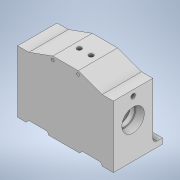
# Autodesk Inventor part: 731113
Saved by Autodesk Inventor 2022 (Build 260153000, 153)
## iProperties
Created: 2021-10-26
Part Number: 731113
Material: Типовые
Document SubType Name: Modeling
Designer: RaNSiD
Density: 1 g/cm^3
Appearance: По умолчанию
Author: RaNSiD
Autodesk Inventor part; units mm, degrees
ref_plane "YZ Plane" through (0, 0, 0) normal (1, 0, 0) x (0, 1, 0)
ref_plane "XZ Plane" through (0, 0, 0) normal (0, 1, 0) x (-1, 0, 0)
ref_plane "XY Plane" through (0, 0, 0) normal (0, 0, 1) x (1, 0, 0)
sketch "Эскиз1" plane through (0, 0, 0) normal (0, 0, 1) x (1, 0, 0)
  line L0 (0, 0) -> (170, 0)
  line L1 (170, 0) -> (170, 110)
  line L2 (170, 110) -> (150, 110)
  line L3 (0, 110) -> (0, 0)
  line L4 (20, 110) -> (62.5, 125.4687)
  line L5 (62.5, 125.4687) -> (107.5, 125.4687)
  line L6 (107.5, 125.4687) -> (150, 110)
  line L7 (20, 110) -> (0, 110)
  dimension "d0" = 170
  dimension "d1" = 110
  dimension "d3" = 45
  dimension "d4" = 160
  dimension "d5" = 160
  dimension "d6" = 20
  constraints: 16 end point, 3 parallel, 2 equal length, 2 horizontal, 1 perpendicular
  measures "d0" distance of L3.start L1.end
  measures "d1" distance of L1.end L0.end
  measures "d3" distance of L4.end L5.end
  measures "d4" angle of L7 L4
  measures "d5" angle of L2 L6
  measures "d6" distance of L4.start L3.start
extrude "Выдавливание1" add sketch "Эскиз1" along normal mid plane 70
sketch "Эскиз2" plane through (0, 0, 35) normal (-1, 0, 0) x (0, 0, 1)
  line L0 (-70, 0) -> (-87, 0)
  line L1 (-87, 0) -> (-87, 10)
  line L2 (-87, 10) -> (-70, 10)
  line L3 (-70, 10) -> (-70, 0)
  point P0 (-35, 0)
  dimension "d9" = 17
  dimension "d10" = 10
  constraints: 8 end point, 2 parallel, 1 horizontal, 1 perpendicular
  measures "d9" distance of L1.end L2.end
  measures "d10" distance of L0.end L1.end
extrude "Выдавливание2" add sketch "Эскиз2" against normal blind 170
fillet "Сопряжение1" radius 7 1 edges at (85, 10, -35)
sketch "Эскиз3" plane through (0, 0, 35) normal (0, 0, 1) x (1, 0, 0)
  line L0 (0, 0) -> (170, 0) construction
  line L1 (20, 0) -> (55, 0)
  line L2 (55, 0) -> (55, 5)
  line L3 (55, 5) -> (20, 5)
  line L4 (20, 5) -> (20, 0)
  line L5 (115, 0) -> (150, 0)
  line L6 (150, 0) -> (150, 5)
  line L7 (150, 5) -> (115, 5)
  line L8 (115, 5) -> (115, 0)
  line L9 (20, 5) -> (0, 5) construction
  line L10 (0, 110) -> (0, 0) construction
  line L11 (115, 5) -> (55, 5) construction
  line L12 (150, 5) -> (170, 5) construction
  line L13 (170, 0) -> (170, 110) construction
  dimension "d14" = 35
  dimension "d15" = 5
  dimension "d16" = 35
  dimension "d17" = 5
  dimension "d18" = 20
  constraints: 22 end point, 5 point on line, 4 parallel, 3 horizontal, 2 perpendicular, 1 collinear
  measures "d14" distance of L3.end L2.end
  measures "d15" distance of L2.end L1.end
  measures "d16" distance of L7.end L6.end
  measures "d17" distance of L6.end L5.end
  measures "d18" distance of L6.end L12.end
extrude "Выдавливание3" cut sketch "Эскиз3" against normal through all
fillet "Сопряжение2" radius 5 2 edges at (150, 5, -8.5) (55, 5, -8.5)
chamfer "Фаска1" distance 5 angle 45 2 edges at (20, 0, -8.5) (115, 0, -8.5)
sketch "Эскиз4" plane through (0, 0, 35) normal (-1, 0, 0) x (0, 0, 1)
  line L0 (0, 110) -> (-70, 110) construction
  point P0 (-35, 0)
  point P1 (-35, 100)
  dimension "d25" = 10
  constraints: 1 vertical alignment
  measures "d25" distance from line of L0 point (-35, 100)
hole "Отверстие1" at (0, 100, 0) direction (1, 0, 0) diameter 8 end through all
sketch "Эскиз5" plane through (62.5, 125.4687, 35) normal (0, 1, 0) x (1, 0, 0)
  line L0 (0, 70) -> (0, 0) construction
  line L1 (45, 70) -> (45, 0) construction
  point P0 (-62.5, 35)
  point P1 (12, 35)
  point P2 (33, 35)
  dimension "d33" = 12
  dimension "d34" = 12
  constraints: 2 horizontal alignment
  measures "d33" distance from line of L0 point (12, 35)
  measures "d34" distance from line of L1 point (33, 35)
hole "Отверстие2" at (74.5, 125.4687, 0) at (95.5, 125.4687, 0) direction (0, -1, 0) diameter 8 depth 34
sketch "Эскиз6" plane through (0, 0, 35) normal (0, 0, 1) x (1, 0, 0)
  line L0 (70.5, 125.4687) -> (78.5, 125.4687) projected
  line L1 (91.5, 125.4687) -> (99.5, 125.4687) projected
  line L2 (0, 96) -> (0, 104) projected
  line L3 (170, 104) -> (170, 96) projected
  line L4 (107.5, 125.4687) -> (62.5, 125.4687) projected
  point P0 (0, 0)
  point P1 (62.5, 119.4687)
  point P2 (107.5, 119.4687)
  dimension "d42" = 6
  constraints: 2 vertical alignment, 1 horizontal alignment
  measures "d42" distance from line of L4 point (107.5, 119.469)
hole "Отверстие3" at (62.5, 119.4687, 35) at (107.5, 119.4687, 35) direction (0, 0, -1) diameter 5 end through all
sketch "Эскиз7" plane through (0, 0, 0) normal (0, 0, 1) x (1, 0, 0)
  line L0 (0, 17) -> (0, 110) construction
  line L1 (0, 63.5) -> (170, 63.5)
  line L2 (170, 110) -> (170, 17) construction
  line L3 (0, 83.5) -> (15, 83.5)
  line L4 (0, 63.5) -> (0, 83.5)
  line L5 (15, 83.5) -> (15, 81.5)
  line L6 (15, 81.5) -> (23, 81.5)
  line L7 (23, 81.5) -> (25, 83.5)
  line L8 (62.5, 125.4687) -> (107.5, 125.4687) construction
  line L9 (55, 0) -> (110, 0) projected
  line L10 (85, 125.4687) -> (85, 0) construction
  line L11 (170, 83.5) -> (155, 83.5)
  line L12 (170, 63.5) -> (170, 83.5)
  line L13 (155, 83.5) -> (155, 81.5)
  line L14 (155, 81.5) -> (147, 81.5)
  line L15 (147, 81.5) -> (145, 83.5)
  line L16 (145, 83.5) -> (145, 78.5)
  line L17 (145, 78.5) -> (142.1716, 75.6716)
  line L18 (142.1716, 75.6716) -> (133.1716, 75.6716)
  line L19 (133.1716, 75.6716) -> (130.3431, 78.5)
  line L20 (130.3431, 78.5) -> (130.3431, 83.5)
  line L21 (130.3431, 83.5) -> (122.3431, 83.5)
  line L22 (145, 83.5) -> (145, 78.5)
  line L23 (145, 78.5) -> (142.1716, 75.6716)
  line L24 (142.1716, 75.6716) -> (133.1716, 75.6716)
  line L25 (133.1716, 75.6716) -> (130.3431, 78.5)
  line L26 (130.3431, 78.5) -> (130.3431, 83.5)
  line L27 (130.3431, 83.5) -> (122.3431, 83.5)
  line L28 (122.3431, 83.5) -> (122.3431, 78.5)
  line L29 (122.3431, 78.5) -> (119.5147, 75.6716)
  line L30 (119.5147, 75.6716) -> (110.5147, 75.6716)
  line L31 (110.5147, 75.6716) -> (107.6863, 78.5)
  line L32 (107.6863, 78.5) -> (107.6863, 83.5)
  line L33 (107.6863, 83.5) -> (99.6863, 83.5)
  line L34 (99.6863, 83.5) -> (99.6863, 78.5)
  line L35 (99.6863, 78.5) -> (96.8579, 75.6716)
  line L36 (96.8579, 75.6716) -> (87.8579, 75.6716)
  line L37 (87.8579, 75.6716) -> (85.0294, 78.5)
  line L38 (85.0294, 78.5) -> (85.0294, 83.5)
  line L39 (85.0294, 83.5) -> (77.0294, 83.5)
  line L40 (77.0294, 83.5) -> (77.0294, 78.5)
  line L41 (77.0294, 78.5) -> (74.201, 75.6716)
  line L42 (74.201, 75.6716) -> (65.201, 75.6716)
  line L43 (65.201, 75.6716) -> (62.3726, 78.5)
  line L44 (62.3726, 78.5) -> (62.3726, 83.5)
  line L45 (62.3726, 83.5) -> (54.3726, 83.5)
  line L46 (62.3726, 83.5) -> (54.3726, 83.5)
  line L47 (62.3726, 78.5) -> (62.3726, 83.5)
  line L48 (65.201, 75.6716) -> (62.3726, 78.5)
  line L49 (74.201, 75.6716) -> (65.201, 75.6716)
  line L50 (77.0294, 78.5) -> (74.201, 75.6716)
  line L51 (77.0294, 83.5) -> (77.0294, 78.5)
  line L52 (39.7157, 83.5) -> (25, 83.5)
  line L53 (39.7157, 78.5) -> (39.7157, 83.5)
  line L54 (42.5442, 75.6716) -> (39.7157, 78.5)
  line L55 (51.5442, 75.6716) -> (42.5442, 75.6716)
  line L56 (54.3726, 78.5) -> (51.5442, 75.6716)
  line L57 (54.3726, 83.5) -> (54.3726, 78.5)
  line L58 (25, 83.5) -> (25, 63.5)
  line L59 (145, 83.5) -> (145, 63.5)
  point P0 (0, 0)
  dimension "d52" = 2
  dimension "d54" = 135
  dimension "d55" = 8
  dimension "d84" = 40
  dimension "d85" = 25
  dimension "d86" = 5
  dimension "d87" = 4
  dimension "d88" = 135
  dimension "d89" = 9
  dimension "d90" = 4
  dimension "d91" = 8
  dimension "d92" = 5
  dimension "d93" = 4
  dimension "d94" = 135
  dimension "d95" = 9
  dimension "d96" = 4
  dimension "d97" = 8
  dimension "d98" = 5
  dimension "d99" = 4
  dimension "d100" = 135
  dimension "d101" = 9
  dimension "d102" = 4
  dimension "d103" = 8
  dimension "d104" = 5
  dimension "d105" = 4
  dimension "d106" = 135
  dimension "d107" = 9
  dimension "d108" = 4
  dimension "d109" = 8
  dimension "d110" = 5
  dimension "d111" = 4
  dimension "d112" = 135
  dimension "d113" = 9
  dimension "d114" = 4
  dimension "d115" = 8
  dimension "d116" = 5
  dimension "d117" = 4
  dimension "d118" = 135
  dimension "d119" = 9
  dimension "d120" = 4
  dimension "d121" = 8
  dimension "d122" = 5
  dimension "d123" = 4
  dimension "d124" = 135
  dimension "d125" = 9
  constraints: 112 end point, 25 perpendicular, 14 parallel, 8 vertical, 5 symmetric about line, 4 point on line, 3 midpoint, 1 horizontal, 1 horizontal alignment
  measures "d52" distance of L3.end L5.end
  measures "d54" angle of L3 L7
  measures "d55" distance of L5.end L6.end
  measures "d84" diameter of L3 L1
  measures "d85" distance of L3.start L7.end
  measures "d86" distance of L15.end L16.end
  measures "d87" distance of L16.end L17.end
  measures "d88" angle of L16 L17
  measures "d89" distance of L17.end L18.end
  measures "d90" distance of L18.end L19.end
  measures "d91" distance of L20.end L21.end
  measures "d92" distance of L15.end L23.start
  measures "d93" distance of L23.start L24.start
  measures "d94" angle of L22 L23
  measures "d95" distance of L24.start L25.start
  measures "d96" distance of L25.start L26.start
  measures "d97" distance of L27.start L27.end
  measures "d98" distance of L21.end L29.start
  measures "d99" distance of L29.start L30.start
  measures "d100" angle of L28 L29
  measures "d101" distance of L30.start L31.start
  measures "d102" distance of L31.start L32.start
  measures "d103" distance of L33.start L33.end
  measures "d104" distance of L33.end L35.start
  measures "d105" distance of L35.start L36.start
  measures "d106" angle of L34 L35
  measures "d107" distance of L36.start L37.start
  measures "d108" distance of L37.start L38.start
  measures "d109" distance of L39.end L39.start
  measures "d110" distance of L39.end L41.start
  measures "d111" distance of L41.start L42.start
  measures "d112" angle of L40 L41
  measures "d113" distance of L42.start L43.start
  measures "d114" distance of L43.start L44.start
  measures "d115" distance of L45.start L45.end
  measures "d116" distance of L39.end L50.start
  measures "d117" distance of L50.start L49.start
  measures "d118" angle of L51 L50
  measures "d119" distance of L49.start L48.start
  measures "d120" distance of L48.start L47.start
  measures "d121" distance of L46.start L46.end
  measures "d122" distance of L45.end L56.start
  measures "d123" distance of L56.start L55.start
  measures "d124" angle of L57 L56
  measures "d125" distance of L55.start L54.start
revolve "Вращение2" cut sketch "Эскиз7" angle 360 about axis through (0, 63.5, 0) along (1, 0, 0) contours L4 L3 L5 L6 L7 L58 L1 | L59 L16 L15 L14 L13 L11 L12 L1
sketch "Эскиз9" plane through (0, 0, 0) normal (0, 0, 1) x (1, 0, 0)
  line L0 (25, 83.5) -> (25, 43.5) construction
  line L1 (25, 43.5) -> (145, 43.5)
  line L2 (145, 43.5) -> (145, 15)
  line L3 (145, 15) -> (91.8199, 15)
  line L4 (25, 15) -> (25, 43.5)
  line L5 (145, 83.5) -> (145, 43.5) construction
  line L6 (50, 5) -> (20, 5) construction
  line L7 (73.1801, 15) -> (75, 10)
  line L8 (75, 10) -> (90, 10)
  line L9 (0, 17) -> (170, 17) construction
  line L10 (90, 10) -> (91.8199, 15)
  line L11 (73.1801, 15) -> (25, 15)
  line L12 (55, 0) -> (110, 0) construction
  point P0 (0, 0)
  point P1 (145, 63.5)
  point P2 (82.5, 10)
  point P3 (82.5, 0)
  dimension "d178" = 110
  dimension "d179" = 110
  dimension "d180" = 15
  dimension "d181" = 5
  dimension "d182" = 10
  constraints: 16 end point, 4 parallel, 3 midpoint, 2 vertical alignment, 1 horizontal, 1 horizontal alignment, 1 perpendicular
  measures "d178" angle of L8 L10
  measures "d179" angle of L8 L7
  measures "d180" distance of L7.end L8.end
  measures "d181" distance between parallel lines of L3 L8
  measures "d182" distance between parallel lines of L6 L11
extrude "Выдавливание4" cut sketch "Эскиз9" along normal mid plane 15
sketch "Эскиз10" plane through (75, 10, -7.5) normal (0, 1, 0) x (1, 0, 0)
  line L0 (15, 0) -> (0, 0) construction
  line L1 (15, 0) -> (15, -15) construction
  point P0 (-75, -7.5)
  point P1 (7.5, -7.5)
  point P2 (7.5, 0)
  point P3 (15, -7.5)
  constraints: 2 midpoint, 1 horizontal alignment, 1 vertical alignment
hole "Отверстие4" at (82.5, 10, 0) direction (0, -1, 0) diameter 12 end through all
sketch "Эскиз11" plane through (0, 0, 0) normal (0, 0, 1) x (1, 0, 0)
  line L0 (0, 17) -> (0, 110) construction
  line L1 (0, 63.5) -> (170, 63.5)
  line L2 (170, 127) -> (170, 0) construction
  line L3 (0, 83.5) -> (15, 83.5)
  line L4 (0, 63.5) -> (0, 83.5)
  line L5 (15, 83.5) -> (15, 81.5)
  line L6 (15, 81.5) -> (23, 81.5)
  line L7 (23, 81.5) -> (25, 83.5)
  line L8 (62.5, 125.4687) -> (107.5, 125.4687) construction
  line L9 (55, 0) -> (110, 0) construction
  line L10 (85, 125.4687) -> (85, 0) construction
  line L11 (147, 81.5) -> (145, 83.5)
  line L12 (155, 81.5) -> (147, 81.5)
  line L13 (155, 83.5) -> (155, 81.5)
  line L14 (170, 83.5) -> (155, 83.5)
  line L15 (170, 63.5) -> (170, 83.5)
  line L16 (145, 83.5) -> (145, 78.5)
  line L17 (145, 78.5) -> (142.1716, 75.6716)
  line L18 (142.1716, 75.6716) -> (133.1716, 75.6716)
  line L19 (133.1716, 75.6716) -> (130.3431, 78.5)
  line L20 (130.3431, 78.5) -> (130.3431, 83.5)
  line L21 (130.3431, 83.5) -> (122.3431, 83.5)
  line L22 (130.3431, 83.5) -> (122.3431, 83.5)
  line L23 (130.3431, 78.5) -> (130.3431, 83.5)
  line L24 (133.1716, 75.6716) -> (130.3431, 78.5)
  line L25 (142.1716, 75.6716) -> (133.1716, 75.6716)
  line L26 (145, 78.5) -> (142.1716, 75.6716)
  line L27 (145, 83.5) -> (145, 78.5)
  line L28 (107.6863, 83.5) -> (99.6863, 83.5)
  line L29 (107.6863, 78.5) -> (107.6863, 83.5)
  line L30 (110.5147, 75.6716) -> (107.6863, 78.5)
  line L31 (119.5147, 75.6716) -> (110.5147, 75.6716)
  line L32 (122.3431, 78.5) -> (119.5147, 75.6716)
  line L33 (122.3431, 83.5) -> (122.3431, 78.5)
  line L34 (85.0294, 83.5) -> (77.0294, 83.5)
  line L35 (85.0294, 78.5) -> (85.0294, 83.5)
  line L36 (87.8579, 75.6716) -> (85.0294, 78.5)
  line L37 (96.8579, 75.6716) -> (87.8579, 75.6716)
  line L38 (99.6863, 78.5) -> (96.8579, 75.6716)
  line L39 (99.6863, 83.5) -> (99.6863, 78.5)
  line L40 (62.3726, 83.5) -> (54.3726, 83.5)
  line L41 (62.3726, 78.5) -> (62.3726, 83.5)
  line L42 (65.201, 75.6716) -> (62.3726, 78.5)
  line L43 (74.201, 75.6716) -> (65.201, 75.6716)
  line L44 (77.0294, 78.5) -> (74.201, 75.6716)
  line L45 (77.0294, 83.5) -> (77.0294, 78.5)
  line L46 (62.3726, 83.5) -> (54.3726, 83.5)
  line L47 (62.3726, 78.5) -> (62.3726, 83.5)
  line L48 (65.201, 75.6716) -> (62.3726, 78.5)
  line L49 (74.201, 75.6716) -> (65.201, 75.6716)
  line L50 (77.0294, 78.5) -> (74.201, 75.6716)
  line L51 (77.0294, 83.5) -> (77.0294, 78.5)
  line L52 (39.7157, 83.5) -> (25, 83.5)
  line L53 (39.7157, 78.5) -> (39.7157, 83.5)
  line L54 (42.5442, 75.6716) -> (39.7157, 78.5)
  line L55 (51.5442, 75.6716) -> (42.5442, 75.6716)
  line L56 (54.3726, 78.5) -> (51.5442, 75.6716)
  line L57 (54.3726, 83.5) -> (54.3726, 78.5)
  line L58 (25, 83.5) -> (25, 51.5)
  line L59 (145, 83.5) -> (145, 51.5)
  line L60 (0, 17) -> (0, 110) projected
  line L61 (62.5, 125.4687) -> (107.5, 125.4687) projected
  line L62 (55, 0) -> (110, 0) projected
  line L63 (0, 51.5) -> (170, 51.5)
  point P0 (170, 110)
  point P1 (82.5, 0)
  dimension "d193" = 2
  dimension "d194" = 135
  dimension "d195" = 8
  dimension "d196" = 40
  dimension "d197" = 25
  dimension "d198" = 5
  dimension "d199" = 4
  dimension "d200" = 135
  dimension "d201" = 9
  dimension "d202" = 4
  dimension "d203" = 8
  dimension "d204" = 5
  dimension "d205" = 4
  dimension "d206" = 135
  dimension "d207" = 9
  dimension "d208" = 4
  dimension "d209" = 8
  dimension "d210" = 5
  dimension "d211" = 4
  dimension "d212" = 135
  dimension "d213" = 9
  dimension "d214" = 4
  dimension "d215" = 8
  dimension "d216" = 5
  dimension "d217" = 4
  dimension "d218" = 135
  dimension "d219" = 9
  dimension "d220" = 4
  dimension "d221" = 8
  dimension "d222" = 5
  dimension "d223" = 4
  dimension "d224" = 135
  dimension "d225" = 9
  dimension "d226" = 4
  dimension "d227" = 8
  dimension "d228" = 5
  dimension "d229" = 4
  dimension "d230" = 135
  dimension "d231" = 9
  dimension "d232" = 4
  dimension "d233" = 8
  dimension "d234" = 5
  dimension "d235" = 4
  dimension "d236" = 135
  dimension "d237" = 9
  dimension "d238" = 12
  constraints: 122 end point, 24 perpendicular, 14 parallel, 10 vertical, 7 midpoint, 6 point on line, 5 coincident, 5 symmetric about line, 4 horizontal alignment, 3 vertical alignment, 1 horizontal
  measures "d193" distance of L3.end L5.end
  measures "d194" angle of L3 L7
  measures "d195" distance of L5.end L6.end
  measures "d196" diameter of L3 L1
  measures "d197" distance of L3.start L7.end
  measures "d198" distance of L11.end L16.end
  measures "d199" distance of L16.end L17.end
  measures "d200" angle of L16 L17
  measures "d201" distance of L17.end L18.end
  measures "d202" distance of L18.end L19.end
  measures "d203" distance of L20.end L21.end
  measures "d204" distance of L11.end L26.start
  measures "d205" distance of L26.start L25.start
  measures "d206" angle of L27 L26
  measures "d207" distance of L25.start L24.start
  measures "d208" distance of L24.start L23.start
  measures "d209" distance of L22.start L22.end
  measures "d210" distance of L21.end L32.start
  measures "d211" distance of L32.start L31.start
  measures "d212" angle of L33 L32
  measures "d213" distance of L31.start L30.start
  measures "d214" distance of L30.start L29.start
  measures "d215" distance of L28.start L28.end
  measures "d216" distance of L28.end L38.start
  measures "d217" distance of L38.start L37.start
  measures "d218" angle of L39 L38
  measures "d219" distance of L37.start L36.start
  measures "d220" distance of L36.start L35.start
  measures "d221" distance of L34.end L34.start
  measures "d222" distance of L34.end L44.start
  measures "d223" distance of L44.start L43.start
  measures "d224" angle of L45 L44
  measures "d225" distance of L43.start L42.start
  measures "d226" distance of L42.start L41.start
  measures "d227" distance of L40.start L40.end
  measures "d228" distance of L34.end L50.start
  measures "d229" distance of L50.start L49.start
  measures "d230" angle of L51 L50
  measures "d231" distance of L49.start L48.start
  measures "d232" distance of L48.start L47.start
  measures "d233" distance of L46.start L46.end
  measures "d234" distance of L40.end L56.start
  measures "d235" distance of L56.start L55.start
  measures "d236" angle of L57 L56
  measures "d237" distance of L55.start L54.start
  measures "d238" distance between parallel lines of L1 L63
revolve "Вращение4" cut sketch "Эскиз11" angle 360 about axis through (0, 51.5, 0) along (1, 0, 0) contours L58 L52 L53 L54 L55 L56 L57 L40 L41 L42 L43 L44 L45 L34 L35 L36 L37 L38 L39 L28 L29 L30 L31 L32 L33 L21 L20 L19 L18 L17 L59 L1 | L1 L59 L63 L58
